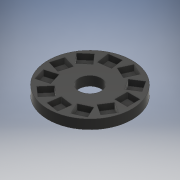
# Autodesk Inventor part: SG01
Saved by Autodesk Inventor 2017 SP1 (Build 210196100, 196)
## iProperties
Created: 2019-09-21
Part Number: SG01
Material: ABS Plastic
Document SubType Name: Modeling
Designer: Dell
Density: 1.06 g/cm^3
Appearance: Smooth - Black
Mass: 48.3343 g
Surface Area: 191.823 cm^2
Volume: 45.5984 cm^3
Author: Dell
Autodesk Inventor part; units mm, degrees
ref_plane "YZ Plane" through (0, 0, 0) normal (1, 0, 0) x (0, 1, 0)
ref_plane "XZ Plane" through (0, 0, 0) normal (0, 1, 0) x (-1, 0, 0)
ref_plane "XY Plane" through (0, 0, 0) normal (0, 0, 1) x (1, 0, 0)
sketch "Sketch1" plane through (0, 0, 0) normal (0, 0, 1) x (1, 0, 0)
  circle A0 centre (0, 0) radius 45
  circle A1 centre (0, 0) radius 12
  dimension "d0" = 90
  dimension "d1" = 24
  constraints: 2 centre point, 2 coincident
  measures "d0" diameter of A0
  measures "d1" diameter of A1
extrude "Extrusion1" add sketch "Sketch1" along normal blind 10
sketch "Sketch2" plane through (0, 0, 10) normal (0, 0, 1) x (1, 0, 0)
  line L0 (27.3, 12.7) -> (40, 12.7)
  line L1 (40, 12.7) -> (40, 0)
  line L2 (40, 0) -> (27.3, 0)
  line L3 (27.3, 0) -> (27.3, 12.7)
  line L4 (40.5, 13.2) -> (26.8, 13.2)
  line L5 (26.8, 13.2) -> (26.8, -0.5)
  line L6 (26.8, -0.5) -> (40.5, -0.5)
  line L7 (40.5, -0.5) -> (40.5, 13.2)
  point P0 (0, 0)
  dimension "d4" = 12.7
  dimension "d5" = 12.7
  dimension "d6" = 40
  dimension "d7" = 0.5
  constraints: 16 end point, 4 parallel, 2 perpendicular, 1 horizontal, 1 horizontal alignment, 3 other
  measures "d4" distance of L1.end L2.end
  measures "d5" distance of L0.end L1.end
  measures "d6" distance of point (0, 0) L1.end
  measures "d7" distance between parallel lines of L0 L4
extrude "Extrusion2" cut sketch "Sketch2" against normal blind 6.35 contours L0 L1 L2 L3 | L7 L6 L5 L4
pattern_circular "Circular Pattern1" count 11 over 360 about axis through (0, 0, 0) along (0, 0, 1) of "Extrusion2"
sketch "Sketch3" plane through (0, 0, 10) normal (0, 0, 1) x (1, 0, 0)
  circle A0 centre (20, 0) radius 1.75
  circle A1 centre (14.1421, 14.1421) radius 1.75
  circle A2 centre (0, 20) radius 1.75
  circle A3 centre (-14.1421, 14.1421) radius 1.75
  circle A4 centre (-20, 0) radius 1.75
  circle A5 centre (-14.1421, -14.1421) radius 1.75
  circle A6 centre (0, -20) radius 1.75
  circle A7 centre (14.1421, -14.1421) radius 1.75
  point P0 (0, 0)
  dimension "d13" = 3.5
  dimension "d14" = 20
  dimension "d17" = 360
  constraints: 8 centre point, 1 horizontal alignment, 17 other
  measures "d13" diameter of A0
  measures "d14" distance of A0.centre point (0, 0)
extrude "Extrusion3" [suppressed]
body "Solid1"
